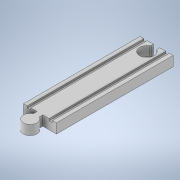
# Autodesk Inventor part: Vasilestraightrack
Saved by Autodesk Inventor 2020 (Build 240168000, 168)
## iProperties
Created: 2020-04-30
Part Number: Vasilestraightrack
Material: Generic
Document SubType Name: Modeling
Designer: al
Density: 1 g/cm^3
Appearance: Default
Author: al
Autodesk Inventor part; units mm, degrees
ref_plane "YZ Plane" through (0, 0, 0) normal (1, 0, 0) x (0, 1, 0)
ref_plane "XZ Plane" through (0, 0, 0) normal (0, 1, 0) x (-1, 0, 0)
ref_plane "XY Plane" through (0, 0, 0) normal (0, 0, 1) x (1, 0, 0)
sketch "Sketch1" plane through (0, 0, 0) normal (0, 0, 1) x (1, 0, 0)
  line L0 (7.2152, 8.367) -> (312.0152, 8.367)
  line L1 (312.0152, 94.727) -> (7.2152, 94.727)
  arc A0 (302.9528, 61.3442) -> (302.9528, 41.7499) centre (286.6152, 51.547) ccw
  line L2 (305.6758, 59.802) -> (312.0152, 59.802)
  line L3 (312.0152, 43.292) -> (305.6758, 43.292)
  line L4 (312.0152, 51.547) -> (337.1565, 51.547) construction
  arc A1 (302.9528, 61.3442) -> (305.6758, 59.802) centre (305.6758, 62.977) ccw
  arc A2 (305.6758, 43.292) -> (302.9528, 41.7499) centre (305.6758, 40.117) ccw
  line L5 (312.0152, 8.367) -> (312.0152, 43.292)
  line L6 (312.0152, 59.802) -> (312.0152, 94.727)
  arc A3 (-2.1204, 59.167) -> (-2.1204, 43.927) centre (-18.1848, 51.547) ccw
  line L7 (7.2152, 43.927) -> (-2.1204, 43.927)
  line L8 (-2.1204, 59.167) -> (7.2152, 59.167)
  line L9 (354.0946, 51.547) -> (-104.1759, 51.547) construction
  line L10 (7.2152, 94.727) -> (7.2152, 59.167)
  line L11 (7.2152, 43.927) -> (7.2152, 8.367)
  point P0 (0, 0)
  point P1 (303.7837, 59.802)
  point P2 (303.7837, 43.292)
  dimension "d0" = 304.8
  dimension "d1" = 86.36
  dimension "d2" = 38.1
  dimension "d4" = 43.18
  dimension "d7" = 3.175
  dimension "d8" = 35.56
  dimension "d10" = 43.18
  dimension "d12" = 7.62
  dimension "d13" = 43.18
  constraints: 24 end point, 10 point on circle, 7 parallel, 5 horizontal, 4 centre point, 4 tangent, 2 perpendicular, 2 point on line, 1 equal radius
  measures "d0" distance of L1.end L1.start
  measures "d1" distance of L1.start L0.end
  measures "d2" diameter of A0
  measures "d4" distance from line of L1 A0.centre
  measures "d7" radius of A1
  measures "d8" diameter of A3
  measures "d10" distance from line of A3.centre L0
  measures "d12" distance between parallel lines of L8 L9
  measures "d13" distance between parallel lines of L0 L9
extrude "Extrusion1" add sketch "Sketch1" along normal blind 25.4
sketch "Sketch2" plane through (7.2152, 8.367, 0) normal (-1, 0, 0) x (0, 0, 1)
  line L0 (0, 35.56) -> (0, 0) projected
  line L1 (0, 0) -> (25.4, 0) projected
  line L2 (25.4, 35.56) -> (25.4, 0) projected
  line L3 (0, 35.56) -> (25.4, 35.56) projected
  line L4 (25.4, 35.56) -> (25.4, 0) projected
  line L5 (25.4, 10.16) -> (20.6375, 10.16)
  line L6 (20.6375, 10.16) -> (20.6375, 19.05)
  line L7 (20.6375, 19.05) -> (25.4, 19.05)
  line L8 (25.4, 19.05) -> (25.4, 10.16)
  point P0 (0, -8.367)
  dimension "d16" = 4.7625
  dimension "d17" = 8.89
  dimension "d18" = 10.16
  constraints: 8 end point, 2 parallel, 1 horizontal, 1 perpendicular, 1 point on line
  measures "d16" distance of L5.start L5.end
  measures "d17" distance of L5.end L6.end
  measures "d18" distance between parallel lines of L1 L5
extrude "Extrusion2" cut sketch "Sketch2" against normal blind 304.8 contours L2 L5 L6 L7
ref_plane "Work Plane1" through (7.2152, 51.547, 0) normal (0, -1, 0) x (1, 0, 0)
mirror "Mirror1" about plane through (7.2152, 51.547, 0) normal (0, -1, 0) of "Extrusion2"
body "Solid1"
